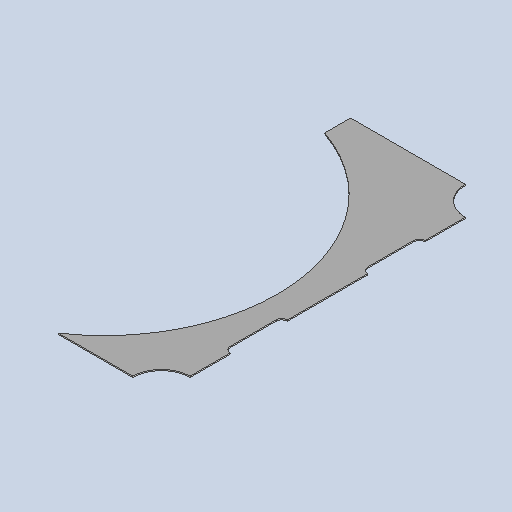
# Autodesk Inventor part: TRM 013 top main
Saved by Autodesk Inventor 2025 (Build 290162010, 162A)
## iProperties
Created: 2024-08-07
Part Number: TRM 013 top main
Material: AISI 304
Document SubType Name: Sheet Metal
Designer: pokla
Density: 8.02768 g/cm^3
Flat Pattern Width: 25 cm
Flat Pattern Length: 58 cm
Flat Pattern Area: 1450 cm^2
Sheet Metal Rule: AISI304 2mm Die16
Sheet Metal Width: 250,000 mm
Sheet Metal Length: 580,000 mm
Sheet Metal Area: 145000,000 mm^2
Appearance: Default
Stock Number: ТРМ 013 верх основное
Mass: 903.946 g
Surface Area: 1160.08 cm^2
Volume: 112.604 cm^3
Author: pokla
Autodesk Inventor part; units mm, degrees
ref_plane "YZ Plane" through (0, 0, 0) normal (1, 0, 0) x (0, 1, 0)
ref_plane "XZ Plane" through (0, 0, 0) normal (0, 1, 0) x (-1, 0, 0)
ref_plane "XY Plane" through (0, 0, 0) normal (0, 0, 1) x (1, 0, 0)
sketch "Sketch1" plane through (0, 0, 0) normal (0, 0, 1) x (1, 0, 0)
  line L0 (-250, -580) -> (0, -580)
  line L1 (0, -580) -> (0, 0)
  line L2 (0, 0) -> (-250, 0)
  line L3 (-250, 0) -> (-250, -580)
  line L4 (-250, -580) -> (0, 0) construction
  line L5 (0, -580) -> (-250, 0) construction
  arc A0 (-180, -580) -> (-250, -45) centre (-349.5833, -330.109) ccw
  circle A1 centre (0, -580) radius 50
  circle A2 centre (0, 0) radius 50
  line L6 (0, -130) -> (0, -210) construction
  line L7 (-10, -130) -> (-10, -210)
  line L8 (10, -210) -> (10, -130)
  arc A3 (10, -130) -> (-10, -130) centre (0, -130) ccw
  arc A4 (-10, -210) -> (10, -210) centre (0, -210) ccw
  line L9 (0, -370) -> (0, -450) construction
  line L10 (-10, -370) -> (-10, -450)
  line L11 (10, -450) -> (10, -370)
  arc A5 (10, -370) -> (-10, -370) centre (0, -370) ccw
  arc A6 (-10, -450) -> (10, -450) centre (0, -450) ccw
  point P0 (0, -170)
  point P1 (0, -410)
  point P2 (0, -120)
  point P3 (0, -50)
  point P4 (-50, 0)
  point P5 (-50, -580)
  point P6 (0, -530)
  point P7 (0, -460)
  point P8 (0, -360)
  point P9 (0, -220)
  dimension "d22" = 580
  dimension "d23" = 250
  dimension "d24" = 302
  dimension "d25" = 45
  dimension "d26" = 180
  dimension "d28" = 100
  dimension "d29" = 20
  dimension "d30" = 80
  dimension "d31" = 170
  dimension "d32" = 170
  measures "d22" distance between parallel lines of L0 L2
  measures "d23" distance between parallel lines of L1 L3
  measures "d24" radius of A0
  measures "d25" distance of L2.end A0.end
  measures "d26" distance of L0.end A0.start
  measures "d28" diameter of A2
  measures "d29" diameter of A4
  measures "d30" distance of L6.end L6.start
  measures "d31" distance of point (0, -170) L1.end
  measures "d32" distance of L0.end point (0, -410)
extrude "Plate1" add sketch "Sketch1" along normal blind 2 contours A0 L3 L2 A2 L1 A3 L7 A4 A5 L10 A6 A1 L0
sketch "Sketch2" plane through (0, 0, 0) normal (0, 0, -1) x (-1, 0, 0)
  line L0 (20, -20) -> (220, -20) construction
  line L1 (220, -20) -> (220, -40) construction
  line L2 (220, -40) -> (20, -40) construction
  line L3 (20, -40) -> (20, -20) construction
  line L4 (50, 0) -> (250, 0) projected
  line L5 (0, -120) -> (0, -50) projected
  point P0 (0, 0)
  point P1 (0, -580)
  point P2 (0, 0)
  dimension "d6" = 200
  dimension "d9" = 20
  dimension "d10" = 20
  dimension "d11" = 20
  constraints: 2 other
  measures "d6" distance of L0.start L0.end
  measures "d9" distance of L0.end L1.end
  measures "d10" distance between parallel lines of L4 L0
  measures "d11" distance between parallel lines of L5 L3
mark "Mark1"
equation "\"d2\" = Thickness"
equation "\"d32\" = d31"
equation "\"BendReliefWidth\" = Thickness"
equation "\"BendReliefDepth\" = 0.5 * Thickness"
equation "\"CornerReliefSize\" = 4 * Thickness"
equation "\"MinimumRemnant\" = 2 * Thickness"
equation "\"TransitionRadius\" = BendRadius"
equation "\"JacobiRadiusSize\" = BendRadius"
equation "\"GapSize\" = Thickness"
equation "\"Thickness\" = 2"
equation "\"BendRadius\" = 2.75"
body "Solid1"
